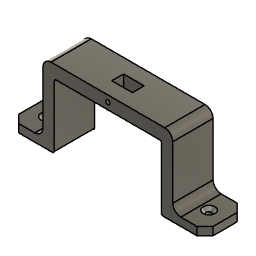
switch holder v8 (Autodesk Fusion 360 design; units mm, degrees)
Autodesk Fusion 360 part; units mm, degrees
sketch "Sketch1" plane through (0, 0, 0) normal (0, 0, 1) x (1, 0, 0)
  line L0 (6.375, 3.625) -> (-6.375, 3.625)
  line L1 (-6.375, 3.625) -> (-6.375, -3.625)
  line L2 (-6.375, -3.625) -> (6.375, -3.625)
  line L3 (6.375, -3.625) -> (6.375, 3.625)
  line L4 (6.375, 3.625) -> (-6.375, -3.625) construction
  line L5 (-6.375, 3.625) -> (6.375, -3.625) construction
  line L6 (33.25, -12.5) -> (-33.25, -12.5)
  line L7 (-33.25, -12.5) -> (-33.25, 12.5)
  line L8 (-33.25, 12.5) -> (33.25, 12.5)
  line L9 (33.25, 12.5) -> (33.25, -12.5)
  line L10 (33.25, -12.5) -> (-33.25, 12.5) construction
  line L11 (-33.25, -12.5) -> (33.25, 12.5) construction
  line L12 (-33.25, -12.5) -> (-40.25, -12.5)
  line L13 (-40.25, -12.5) -> (-40.25, 12.5)
  line L14 (-40.25, 12.5) -> (-33.25, 12.5)
  line L15 (-33.25, 12.5) -> (-33.25, -12.5)
  line L16 (0, 1.75) -> (0, 22.5)
  line L17 (40.25, -12.5) -> (40.25, 12.5)
  line L18 (40.25, 12.5) -> (33.25, 12.5)
  line L19 (33.25, -12.5) -> (33.25, 12.5)
  line L20 (33.25, -12.5) -> (40.25, -12.5)
  dimension "d1" = 12.75
  dimension "d2" = 7.25
  dimension "d3" = 25
  dimension "d4" = 66.5
  dimension "d7" = 7
  dimension "d8" = 25
  constraint horizontal L0
  constraint perpendicular L0 L1
  constraint parallel L0 L2
  constraint parallel L1 L3
  constraint coincident L4 origin
  constraint coincident L5 origin
  constraint horizontal L6
  constraint perpendicular L6 L7
  constraint parallel L6 L8
  constraint parallel L7 L9
  constraint coincident L10 origin
  constraint coincident L11 origin
  constraint horizontal L12
  constraint vertical L13
  constraint horizontal L14
  constraint vertical L15
  constraint symmetric L6.end L16 L6.start
  constraint symmetric L7.end L16 L8.end
  constraint symmetric L12.end L16 L17.start
  constraint symmetric L13.end L16 L17.end
  measures "d1" distance of L1.end L2.end
  measures "d2" distance of L0.end L1.end
  measures "d3" distance of L6.end L7.end
  measures "d4" distance of L7.end L8.end
  measures "d7" distance of L6.end L12.end
  measures "d8" distance of L12.end L13.end
extrude "Extrude1" add sketch "Sketch1" along normal blind 8 contours L6 L7 L8 L9 L15 L19
extrude "Extrude2" add sketch "Sketch1" along normal blind 48 contours L9 L17 L18 L19 L20 | L7 L12 L13 L14 L15
sketch "Sketch2" plane through (0, 0, 48) normal (0, 0, 1) x (-1, 0, 0)
  line L0 (33.25, -12.5) -> (40.25, -12.5)
  line L1 (40.25, -12.5) -> (40.25, 12.5)
  line L2 (40.25, 12.5) -> (33.25, 12.5)
  line L3 (33.25, 12.5) -> (33.25, -12.5)
  line L4 (40.25, 12.5) -> (60.25, 12.5)
  line L5 (60.25, 12.5) -> (60.25, -12.5)
  line L6 (60.25, -12.5) -> (40.25, -12.5)
  line L7 (40.25, -12.5) -> (40.25, 12.5)
  circle A0 centre (50.25, 0) radius 1.7
  line L8 (60.25, 0) -> (40.25, 0)
  line L9 (0, -1.75) -> (0, -22.5)
  line L10 (-60.25, 12.5) -> (-60.25, -12.5)
  line L11 (-60.25, -12.5) -> (-40.25, -12.5)
  line L12 (-40.25, -12.5) -> (-40.25, 12.5)
  line L13 (-40.25, 12.5) -> (-60.25, 12.5)
  line L14 (-60.25, 0) -> (-40.25, 0)
  circle A1 centre (-50.25, 0) radius 1.7
  dimension "d11" = 20
  dimension "d12" = 3.4
  dimension "d13" = 25
  constraint horizontal L4
  constraint vertical L5
  constraint horizontal L6
  constraint vertical L7
  constraint coincident L1.end L2.start
  constraint midpoint L5 L8.start
  constraint midpoint L7 L8.end
  constraint midpoint A0.centre L8
  constraint symmetric L1.end L9 L12.end
  constraint symmetric L4.end L9 L10.start
  constraint symmetric L5.end L9 L10.end
  constraint symmetric L0.end L9 L11.end
  constraint symmetric A0 L9 A1
  constraint symmetric L8.start L9 L14.start
  constraint symmetric L8.end L9 L14.end
  measures "d11" distance of L1.end L4.end
  measures "d12" diameter of A0
  measures "d13" distance of L4.end L5.end
extrude "Extrude3" add sketch "Sketch2" against normal blind 5 contours L1 L5 L6 L7 A0 L8 | L1 L4 L5 L7 A0 L8 | L10 L12 L13 L14 A1 | L10 L11 L12 L14 A1
chamfer "Chamfer1" distance 2 angle 45 2 edges at (-48.665, 0.6147, 43) (51.835, 0.6147, 43)
fillet "Fillet3" radius 5 4 edges at (40.25, 0, 0) (-40.25, 0, 0) (-40.25, 0, 43) (40.25, 0, 43)
fillet "Fillet4" radius 1 4 edges at (-33.25, 0, 8) (33.25, 0, 8) (33.25, 0, 48) (-33.25, 0, 48)
chamfer "Chamfer2" distance 5 angle 45 4 edges at (-60.25, 12.5, 45.5) (-60.25, -12.5, 45.5) (60.25, -12.5, 45.5) (60.25, 12.5, 45.5)
sketch "Sketch3" plane through (0, -12.5, 0) normal (0, -1, 0) x (1, 0, 0)
  line L0 (55.25, 43) -> (55.25, 48)
  line L1 (55.25, 48) -> (34.25, 48)
  arc A0 (34.25, 48) -> (33.25, 47) centre (34.25, 47) ccw
  line L2 (33.25, 47) -> (33.25, 9)
  arc A1 (32.25, 8) -> (33.25, 9) centre (32.25, 9) ccw
  line L3 (32.25, 8) -> (-32.25, 8)
  arc A2 (-33.25, 9) -> (-32.25, 8) centre (-32.25, 9) ccw
  line L4 (-33.25, 9) -> (-33.25, 47)
  arc A3 (-33.25, 47) -> (-34.25, 48) centre (-34.25, 47) ccw
  line L5 (-34.25, 48) -> (-55.25, 48)
  line L6 (-55.25, 48) -> (-55.25, 43)
  line L7 (-55.25, 43) -> (-45.25, 43)
  arc A4 (-40.25, 38) -> (-45.25, 43) centre (-45.25, 38) ccw
  line L8 (-40.25, 38) -> (-40.25, 5)
  arc A5 (-40.25, 5) -> (-35.25, 0) centre (-35.25, 5) ccw
  line L9 (-35.25, 0) -> (35.25, 0)
  arc A6 (35.25, 0) -> (40.25, 5) centre (35.25, 5) ccw
  line L10 (40.25, 5) -> (40.25, 38)
  arc A7 (45.25, 43) -> (40.25, 38) centre (45.25, 38) ccw
  line L11 (45.25, 43) -> (55.25, 43)
  line L12 (-6.375, 0) -> (6.375, 0)
  line L13 (6.375, 0) -> (6.375, 8)
  line L14 (6.375, 8) -> (-6.375, 8)
  line L15 (-6.375, 8) -> (-6.375, 0)
  line L16 (0, 4) -> (0, 0) construction
  line L17 (0, 4) -> (-6.375, 4) construction
  circle A8 centre (0, 4) radius 1.3
  dimension "d39" = 2.6
  constraint coincident L16.end origin
  constraint perpendicular L9 L16
  constraint midpoint L15 L17.end
  constraint perpendicular L15 L17
  constraint coincident L16.start L17.start
  measures "d39" diameter of A8
extrude "Extrude4" cut sketch "Sketch3" against normal blind 8.875 contours A8
equation "d3 = thickness"
equation "d8 = d3"
equation "d13 = thickness"
equation "thickness = 25 mm"
